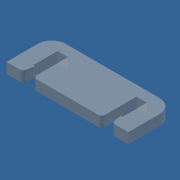
# Autodesk Inventor part: link
Saved by Autodesk Inventor 2014 (Build 180170000, 170)
## iProperties
Created: 2014-02-13
Part Number: link
Material: Glass
Document SubType Name: Sheet Metal
Designer: Lefo
Density: 2.18 g/cm^3
Sheet Metal Rule: Default
Appearance: Clear
Thickness: 0.500 mm
BendRadius: 0.500 mm
BendReliefWidth: 0.500 mm
BendReliefDepth: 0.250 mm
CornerReliefSize: 2.000 mm
MinimumRemnant: 1.000 mm
TransitionRadius: 0.500 mm
JacobiRadiusSize: 0.500 mm
GapSize: 0.500 mm
d0: 35.000 mm
d1: 13.000 mm
d2: 3.000 mm
d3: 0.00 deg
d4: 4.000 mm
d6: 9.850 mm
d7: 3.000 mm
d9: 3.000 mm
d10: 10.000 mm
d15: 9.40 deg
d16: 10.000 mm
d18: 0.00 deg
d19: 1.000 mm
Author: Lefo
Autodesk Inventor part; units mm, degrees
ref_plane "YZ Plane" through (0, 0, 0) normal (1, 0, 0) x (0, 1, 0)
ref_plane "XZ Plane" through (0, 0, 0) normal (0, 1, 0) x (-1, 0, 0)
ref_plane "XY Plane" through (0, 0, 0) normal (0, 0, 1) x (1, 0, 0)
sketch "Sketch1" plane through (0, 0, 0) normal (0, 1, 0) x (-1, 0, 0)
  line L0 (17.5, 6.5) -> (-17.5, 6.5)
  line L1 (-17.5, 6.5) -> (-17.5, -6.5)
  line L2 (-17.5, -6.5) -> (17.5, -6.5)
  line L3 (17.5, -6.5) -> (17.5, 6.5)
  line L4 (17.5, 6.5) -> (-17.5, -6.5) construction
  line L5 (-17.5, 6.5) -> (17.5, -6.5) construction
  point P0 (0, 0)
  dimension "d0" = 35
  dimension "d1" = 13
  constraints: 12 end point, 2 midpoint, 2 parallel, 1 horizontal, 1 perpendicular
  measures "d0" distance of L2.end L1.end
  measures "d1" distance of L1.end L0.end
extrude "Extrusion1" add sketch "Sketch1" along normal blind 3
fillet "Fillet1" radius 4 2 edges at (-17.5, 1.5, -6.5) (17.5, 1.5, -6.5)
sketch "Sketch2" plane through (0, 3, 0) normal (0, 1, 0) x (1, 0, 0)
  line L0 (13.5, 6.5) -> (-13.5, 6.5) projected
  arc A0 (-13.5, 6.5) -> (-17.5, 2.5) centre (-13.5, 2.5) ccw projected
  line L1 (-17.5, -6.5) -> (17.5, -6.5) projected
  line L2 (17.5, -6.5) -> (17.5, 2.5) projected
  line L3 (-9.85, 3.5) -> (-12.85, 3.5)
  line L4 (-12.85, 3.5) -> (-12.85, -6.5)
  line L5 (-12.85, -6.5) -> (-9.85, -6.5)
  line L6 (-9.85, -6.5) -> (-9.85, 3.5)
  line L7 (-9.85, 3.5) -> (-12.85, -6.5) construction
  line L8 (-12.85, 3.5) -> (-9.85, -6.5) construction
  line L9 (0, 6.5) -> (0, -6.5) construction
  line L10 (0, 0) -> (17.5, 0) construction
  line L11 (-11.35, 6.5) -> (-11.35, -3.5) construction
  line L12 (-12.85, -3.5) -> (-12.3536, -3.5)
  line L13 (-12.3536, -3.5) -> (-12.85, -6.5)
  line L14 (9.85, 3.5) -> (12.85, 3.5)
  line L15 (12.85, 3.5) -> (12.85, -6.5)
  line L16 (12.85, -6.5) -> (9.85, -6.5)
  line L17 (9.85, -6.5) -> (9.85, 3.5)
  line L18 (9.85, 3.5) -> (12.85, -6.5) construction
  line L19 (12.85, 3.5) -> (9.85, -6.5) construction
  line L20 (12.85, -3.5) -> (12.3536, -3.5)
  line L21 (12.3536, -3.5) -> (12.85, -6.5)
  point P0 (-11.35, -1.5)
  point P1 (13.5, 2.5)
  point P2 (11.35, -1.5)
  point P3 (11.35, -3.5)
  dimension "d6" = 9.85
  dimension "d7" = 3
  dimension "d9" = 3
  dimension "d10" = 10
  dimension "d15" = 9.396
  dimension "d16" = 10
  constraints: 38 end point, 9 symmetric about line, 6 midpoint, 4 perpendicular, 4 point on line, 2 parallel, 1 collinear, 1 horizontal, 1 vertical alignment
  measures "d6" distance between parallel lines of L9 L6
  measures "d7" distance of L3.start L3.end
  measures "d9" distance between parallel lines of L0 L3
  measures "d10" distance of L11.start L11.end
  measures "d15" angle of L2 L13
  measures "d16" distance between parallel lines of L12 L0
extrude "Extrusion2" cut sketch "Sketch2" against normal up to next contours L13 L12 L4 L3 L6 L1 | L17 L14 L15 L20 L21 L1
fillet "Fillet2" radius 1 4 edges at (-12.85, 1.5, 6.5) (-9.85, 1.5, 6.5) (9.85, 1.5, 6.5) (12.85, 1.5, 6.5)
equation "\"BendRadius\" = Thickness"
equation "\"BendReliefWidth\" = Thickness"
equation "\"BendReliefDepth\" = 0.5 * Thickness"
equation "\"CornerReliefSize\" = 4 * Thickness"
equation "\"MinimumRemnant\" = 2 * Thickness"
equation "\"TransitionRadius\" = BendRadius"
equation "\"JacobiRadiusSize\" = Thickness"
equation "\"GapSize\" = Thickness"
equation "\"Thickness\" = 0.5"
body "Solid1"
